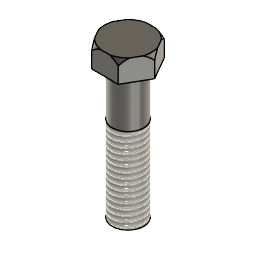
Cap (Autodesk Fusion 360 archive; units mm, degrees)
design "Screw"
Autodesk Fusion 360 part; units mm, degrees
sketch "Sketch1" plane through (0, 0, 0) normal (0, 0, 1) x (1, 0, 0)
  circle A0 centre (0, 0) radius 4.7625
  dimension "d1" = 9.525
  constraint coincident A0.centre origin
  measures "d1" diameter of A0
extrude "Extrude1" add sketch "Sketch1" along normal blind 25.4 makes body 1
thread "Thread1" "ANSI Unified Screw Threads 0.375 3/8-16 UNC 3/8-16 UNC 3A" major diameter 9.4056 minor diameter 7.6327 pitch 1.5875 angle 60 resizes the face on face at (4.7388, -0.4742, 16.9333) on bodies 1
sketch "Sketch2" plane through (0, 0, 25.4) normal (0, 0, 1) x (-1, 0, 0)
  circle A0 centre (0, 0) radius 4.7028
  circle A1 centre (0, 0) radius 4.7625
  dimension "d6" = 9.525
  constraint coincident A0.centre A1.centre
  measures "d6" diameter of A1
extrude "Extrude2" add sketch "Sketch2" along normal blind 14.2875 separate body contours A0 makes body 2
sketch "Sketch3" plane through (0, 0, 39.6875) normal (0, 0, 1) x (-1, 0, 0)
  circle A0 centre (0, 0) radius 4.7028
  circle A1 centre (0, 0) radius 7.9375
  line L0 (-7.9375, 0) -> (-3.9688, -6.8741)
  line L1 (-3.9688, -6.8741) -> (3.9687, -6.8741)
  line L2 (3.9687, -6.8741) -> (7.9375, 0)
  line L3 (7.9375, 0) -> (3.9688, 6.8741)
  line L4 (3.9688, 6.8741) -> (-3.9687, 6.8741)
  line L5 (-3.9687, 6.8741) -> (-7.9375, 0)
  dimension "d9" = 15.875
  constraint coincident A0.centre A1.centre
  constraint coincident A1 L0.start
  measures "d9" diameter of A1
extrude "Extrude3" add sketch "Sketch3" along normal blind 6.35 contours A0 | L0 L1 L2 L3 L4 L5 bodies 2
sketch "Sketch4" plane through (0, 0, 0) normal (0, 1, 0) x (1, 0, 0)
  line L0 (-7.021, -39.6875) -> (-7.9375, -41.275)
  line L1 (-7.9375, -39.6875) -> (-7.9375, -46.0375)
  line L2 (-7.9375, -39.6875) -> (-3.9688, -39.6875)
  line L3 (-7.021, -46.0375) -> (-7.9375, -44.45)
  line L4 (-7.9375, -46.0375) -> (-3.9688, -46.0375)
  line L5 (-7.9375, -46.0375) -> (-7.021, -46.0375)
  line L6 (-7.9375, -46.0375) -> (-7.9375, -44.45)
  line L7 (-7.9375, -39.6875) -> (-7.9375, -41.275)
  line L8 (-7.9375, -39.6875) -> (-7.021, -39.6875)
  dimension "d12" = 1.5875
  dimension "d13" = 150
  dimension "d14" = 1.5875
  dimension "d15" = 150
  constraint coincident L0.end L1
  constraint coincident L0.start L2
  constraint coincident L3.start L4
  constraint coincident L1 L3.end
  constraint coincident L1.end L4.start
  constraint coincident L1.start L2.start
  measures "d12" distance of L0.end L1.start
  measures "d13" angle of L0 L1
  measures "d14" distance of L1.end L3.end
  measures "d15" angle of L1 L3
revolve "Revolve1" cut sketch "Sketch4" angle 360 about axis through (0, 0, 25.4) along (0, 0, -1) contours L1 L3 L4 L5 L6 bodies 2
equation "d9 = ( 5 / 8 ) * 1 in"

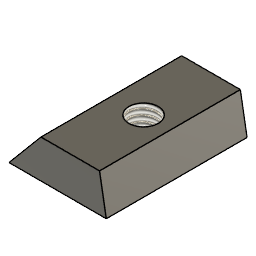
design "Wedge"
Autodesk Fusion 360 part; units mm, degrees
ref_plane "WorkPlane1" through (0, 0, 0.4062) normal (0, 0, 1) x (1, 0, 0)
sketch "Sketch1" plane through (0, 0, 0.4062) normal (0, 0, 1) x (1, 0, 0)
  line L0 (0, 0) -> (0.625, 0)
  line L1 (0.625, 0) -> (0.625, 1.5)
  line L2 (0.625, 1.5) -> (0, 1.5)
  line L3 (0, 1.5) -> (0, 0)
  dimension "d2" = 0.625
  dimension "d3" = 1.5
  constraint horizontal L0
  constraint vertical L1
  constraint horizontal L2
  constraint vertical L3
  constraint coincident L0.start L3.end
  measures "d2" distance of L0.start L0.end
  measures "d3" distance of L0.start L2.end
sketch "Sketch2" plane through (0, 0, 0) normal (0, 1, 0) x (1, 0, 0)
  line L0 (0, 0) -> (0, -0.4062)
  line L1 (0, -0.4062) -> (-0.3409, 0)
  line L2 (0, -0.4062) -> (-0.632, -0.4062) construction
  line L3 (-0.3409, 0) -> (-0.21, 0)
  line L4 (0, -0.4062) -> (0.625, -0.4062)
  line L5 (0.625, -0.4062) -> (0.6966, 0)
  line L6 (0.6966, 0) -> (0, 0)
  line L7 (0, 0) -> (-0.3409, 0)
  dimension "d4" = 0.4063
  dimension "d5" = 50
  dimension "d6" = 0.625
  dimension "d7" = 80
  constraint coincident L0.start L6.end
  constraint vertical L0
  constraint horizontal L2
  constraint perpendicular L0 L3
  constraint perpendicular L0 L4
  measures "d4" distance of L0.start L0.end
  measures "d5" angle of L1 L2
  measures "d6" distance of L0.end L4.end
  measures "d7" angle of L4 L5
extrude "Extrude1" add sketch "Sketch2" along normal blind 1.5
hole "Hole1" at (0.3438, 0.75, 0.4062) direction (0, 0, -1) diameter 0.375 depth 0.41 tip angle 180
scale "Scale1" factor 25.4 about (0, 0, 0.4062) bodies 1
thread "Thread2" "ANSI Unified Screw Threads 0.375 3/8-16 UNC 3/8-16 UNC 3B" major diameter 9.525 minor diameter 7.94 pitch 1.5875 angle 60 resizes the face on face at (9.2054, 14.3112, -6.4728)

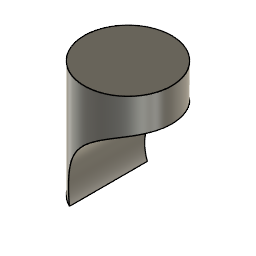
design "Cushion"
Autodesk Fusion 360 part; units mm, degrees
sketch "Sketch1" plane through (0, 0, 0) normal (0, 0, 1) x (1, 0, 0)
  circle A0 centre (0, 0) radius 3.5719
  dimension "d1" = 7.1437
  constraint coincident A0.centre origin
  measures "d1" diameter of A0
extrude "Extrude1" add sketch "Sketch1" along normal blind 9.525
sketch "Sketch2" plane through (0, 0, 0) normal (0, 1, 0) x (1, 0, 0)
  circle A0 centre (3.81, -1.27) radius 5.5563
  dimension "d4" = 11.1125
  measures "d4" diameter of A0
extrude "Extrude2" cut sketch "Sketch2" along normal blind 12.7 and the other way blind 12.7
equation "d1 = ( 9 / 32 ) * 1 in"
equation "d2 = ( 3 / 8 ) * 1 in"
equation "d4 = ( 7 / 16 ) * 1 in"

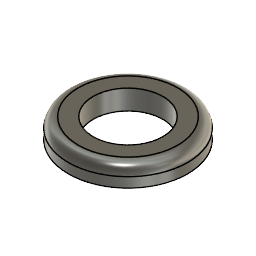
design "Washer"
Autodesk Fusion 360 part; units mm, degrees
sketch "Sketch1" plane through (0, 0, 0) normal (0, 0, 1) x (1, 0, 0)
  circle A0 centre (0, 0) radius 9.525
  dimension "d1" = 19.05
  constraint coincident A0.centre origin
  measures "d1" diameter of A0
extrude "Extrude1" add sketch "Sketch1" along normal blind 3.175
fillet "Fillet1" radius 1.5875 1 edges at (-8.8804, -3.4444, 3.175)
sketch "Sketch2" plane through (0, 0, 3.175) normal (0, 0, 1) x (-1, 0, 0)
  circle A0 centre (0, 0) radius 7.9375
  circle A1 centre (0, 0) radius 5.5563
  dimension "d6" = 11.1125
  constraint coincident A0.centre A1.centre
  measures "d6" diameter of A1
extrude "Extrude2" cut sketch "Sketch2" against normal blind 3.175 contours A1

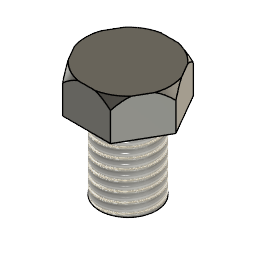
design "Set Screw"
Autodesk Fusion 360 part; units mm, degrees
sketch "Sketch1" plane through (0, 0, 0) normal (0, 0, 1) x (1, 0, 0)
  circle A0 centre (0, 0) radius 4.7625
  dimension "d1" = 9.525
  constraint coincident A0.centre origin
  measures "d1" diameter of A0
extrude "Extrude1" add sketch "Sketch1" along normal blind 12.7
thread "Thread1" "ANSI Unified Screw Threads 0.375 3/8-16 UNC 3/8-16 UNC 3A" major diameter 9.4056 minor diameter 7.6327 pitch 1.5875 angle 60 resizes the face on face at (4.7388, -0.4742, 8.4667)
sketch "Sketch2" plane through (0, 0, 12.7) normal (0, 0, 1) x (-1, 0, 0)
  circle A0 centre (0, 0) radius 4.7028
  circle A1 centre (0, 0) radius 7.9375
  line L0 (-7.9375, 0) -> (-3.9688, -6.8741)
  line L1 (-3.9688, -6.8741) -> (3.9687, -6.8741)
  line L2 (3.9687, -6.8741) -> (7.9375, 0)
  line L3 (7.9375, 0) -> (3.9688, 6.8741)
  line L4 (3.9688, 6.8741) -> (-3.9687, 6.8741)
  line L5 (-3.9687, 6.8741) -> (-7.9375, 0)
  dimension "d6" = 15.875
  constraint coincident A0.centre A1.centre
  constraint coincident A1 L0.start
  measures "d6" diameter of A1
extrude "Extrude2" add sketch "Sketch2" along normal blind 6.35 contours A0 | L0 L1 L2 L3 L4 L5
sketch "Sketch5" plane through (0, 0, 0) normal (0, 1, 0) x (1, 0, 0)
  line L0 (-7.021, -19.05) -> (-7.9375, -17.4625)
  line L1 (-7.9375, -12.7) -> (-7.9375, -19.05)
  line L2 (-7.9375, -19.05) -> (-3.9688, -19.05)
  dimension "d13" = 1.5875
  dimension "d14" = 150
  constraint coincident L0.end L1
  constraint coincident L0.start L2
  measures "d13" distance of L0.end L1.end
  measures "d14" angle of L0 L1
revolve "Revolve1" cut sketch "Sketch5" angle 360 about axis through (0, 0, 0) along (0, 0, -1)
